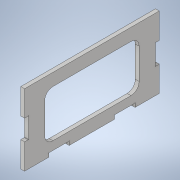
# Autodesk Inventor part: open_case
Saved by Autodesk Inventor 2020 (Build 240168000, 168)
## iProperties
Created: 2019-12-18
Part Number: open_case
Material: Generic
Document SubType Name: Modeling
Designer: fabfarm
Density: 1 g/cm^3
Appearance: Default
Author: fabfarm
Autodesk Inventor part; units mm, degrees
ref_plane "YZ Plane" through (0, 0, 0) normal (1, 0, 0) x (0, 1, 0)
ref_plane "XZ Plane" through (0, 0, 0) normal (0, 1, 0) x (-1, 0, 0)
ref_plane "XY Plane" through (0, 0, 0) normal (0, 0, 1) x (1, 0, 0)
sketch "Sketch1" plane through (0, 0, 0) normal (1, 0, 0) x (0, 1, 0)
  line L0 (-175, -330) -> (175, -330)
  line L1 (175, -330) -> (175, 330)
  line L2 (175, 330) -> (-175, 330)
  line L3 (-175, 330) -> (-175, -330)
  line L4 (-175, -330) -> (175, 330) construction
  line L5 (175, -330) -> (-175, 330) construction
  point P0 (0, 0)
  dimension "d0" = 660
  dimension "d1" = 350
  constraints: 12 end point, 2 midpoint, 2 parallel, 1 horizontal, 1 perpendicular
  measures "d0" distance of L0.end L1.end
  measures "d1" distance of L0.start L0.end
extrude "Extrusion1" add sketch "Sketch1" along normal blind 18.55
sketch "Sketch2" plane through (18.55, 0, 0) normal (1, 0, 0) x (0, 0, -1)
  line L0 (-330, 175) -> (-330, -175) projected
  line L1 (-330, 50.1) -> (-311.45, 50.1)
  line L2 (-311.45, 50.1) -> (-311.45, -50.1)
  line L3 (-311.45, -50.1) -> (-330, -50.1)
  line L4 (-330, -50.1) -> (-330, 50.1)
  line L5 (330, 175) -> (-330, 175) projected
  line L6 (-330, -175) -> (330, -175) projected
  dimension "d20" = 100.2
  dimension "d21" = 124.9
  dimension "d22" = 124.9
  dimension "d23" = 18.55
  constraints: 8 end point, 2 parallel, 1 horizontal, 1 perpendicular, 1 point on line
  measures "d20" distance of L1.end L2.end
  measures "d21" distance from line of L5 L1.end
  measures "d22" distance between parallel lines of L6 L3
  measures "d23" distance of L1.start L1.end
extrude "Extrusion2" cut sketch "Sketch2" against normal blind 18.55
mirror "Mirror1" about plane through (0, 0, 0) normal (0, 0, 1) of "Extrusion2"
sketch "Sketch3" plane through (18.55, 0, 0) normal (1, 0, 0) x (0, 0, -1)
  line L0 (191.45, -115) -> (-191.45, -115)
  line L1 (-231.45, -75) -> (-231.45, 75)
  line L2 (-191.45, 115) -> (191.45, 115)
  line L3 (231.45, 75) -> (231.45, -75)
  line L4 (231.45, -115) -> (-231.45, 115) construction
  line L5 (-231.45, -115) -> (231.45, 115) construction
  line L6 (-330, 115) -> (-311.45, 115) projected
  line L7 (-311.45, -125) -> (-311.45, -145) projected
  arc A0 (-191.45, 115) -> (-231.45, 75) centre (-191.45, 75) ccw
  arc A1 (-231.45, -75) -> (-191.45, -115) centre (-191.45, -75) ccw
  arc A2 (231.45, 75) -> (191.45, 115) centre (191.45, 75) ccw
  arc A3 (191.45, -115) -> (231.45, -75) centre (191.45, -75) ccw
  point P0 (0, 0)
  dimension "d16" = 80
  dimension "d17" = 40
  constraints: 12 end point, 8 point on circle, 8 point on line, 8 tangent, 4 centre point, 3 equal radius, 2 midpoint, 2 parallel, 1 collinear, 1 horizontal, 1 perpendicular
  measures "d16" distance between parallel lines of L7 L1
  measures "d17" radius of A0
extrude "Extrusion3" cut sketch "Sketch3" against normal blind 18.55
sketch "Esquisse4" plane through (18.55, 0, 0) normal (1, 0, 0) x (0, 0, -1)
  line L0 (-311.45, -50.1) -> (-311.45, 50.1) projected
  circle A0 centre (-311.45, 50.1) radius 1.5875
  circle A1 centre (-311.45, -50.1) radius 1.5875
  line L1 (311.45, 50.1) -> (311.45, -50.1) projected
  circle A2 centre (311.45, 50.1) radius 1.5875
  circle A3 centre (311.45, -50.1) radius 1.5875
  point P0 (0, 0)
  dimension "d24" = 3.175
  constraints: 4 centre point, 3 equal radius, 2 coincident
  measures "d24" diameter of A0
extrude "Extrusion4" cut sketch "Esquisse4" against normal blind 18.55
sketch "Esquisse5" plane through (18.55, 0, 0) normal (1, 0, 0) x (0, 0, -1)
  line L0 (-211.5, -175) -> (-111.4, -175)
  line L1 (-111.4, -175) -> (-111.4, -156.35)
  line L2 (-111.4, -156.35) -> (-211.5, -156.35)
  line L3 (-211.5, -156.35) -> (-211.5, -175)
  line L4 (111.4, -175) -> (211.5, -175)
  line L5 (211.5, -175) -> (211.5, -156.35)
  line L6 (211.5, -156.35) -> (111.4, -156.35)
  line L7 (111.4, -156.35) -> (111.4, -175)
  line L8 (-330, -50.1) -> (-330, -175) projected
  line L9 (330, -175) -> (330, -50.1) projected
  line L10 (191.45, -115) -> (-191.45, -115) projected
  point P0 (0, 0)
  dimension "d27" = 100.1
  dimension "d28" = 100.1
  dimension "d29" = 118.5
  dimension "d30" = 118.5
  dimension "d37" = 41.35
  dimension "d38" = 18.65
  constraints: 16 end point, 4 parallel, 2 horizontal, 2 perpendicular, 1 collinear, 1 point on line
  measures "d27" distance of L1.end L2.end
  measures "d28" distance of L5.end L6.end
  measures "d29" distance between parallel lines of L8 L3
  measures "d30" distance between parallel lines of L9 L5
  measures "d37" distance between parallel lines of L10 L2
  measures "d38" distance of L0.end L1.end
extrude "Extrusion5" cut sketch "Esquisse5" against normal blind 20
sketch "Esquisse6" plane through (18.55, 0, 0) normal (1, 0, 0) x (0, 0, -1)
  line L0 (-211.5, -156.35) -> (-111.4, -156.35) projected
  circle A0 centre (-211.5, -156.35) radius 1.6
  circle A1 centre (-111.4, -156.35) radius 1.6
  line L1 (111.4, -156.35) -> (211.5, -156.35) projected
  circle A2 centre (111.4, -156.35) radius 1.6
  line L2 (211.5, -156.35) -> (211.5, -175) projected
  circle A3 centre (211.5, -156.35) radius 1.6
  point P0 (0, 0)
  dimension "d34" = 3.2
  constraints: 4 centre point, 3 equal radius, 2 coincident
  measures "d34" diameter of A1
extrude "Extrusion6" cut sketch "Esquisse6" against normal blind 20
body "Solid1"
